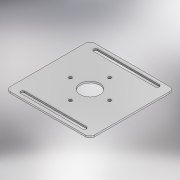
# Autodesk Inventor part: BaseTopPlate
Saved by Autodesk Inventor 2020.3 (Build 243373000, 373)
## iProperties
Created: 2021-08-02
Part Number: BaseTopPlate
Material: Aluminum
Document SubType Name: Modeling
Designer: justi
Density: 2.7 g/cm^3
Appearance: Aluminum - Polished
Author: justi
Autodesk Inventor part; units mm, degrees
ref_plane "YZ Plane" through (0, 0, 0) normal (1, 0, 0) x (0, 1, 0)
ref_plane "XZ Plane" through (0, 0, 0) normal (0, 1, 0) x (-1, 0, 0)
ref_plane "XY Plane" through (0, 0, 0) normal (0, 0, 1) x (1, 0, 0)
sketch "Sketch1" plane through (0, 0, 0) normal (0, 1, 0) x (-1, 0, 0)
  line L0 (-75, -75) -> (75, -75)
  line L1 (75, -75) -> (75, 75)
  line L2 (75, 75) -> (-75, 75)
  line L3 (-75, 75) -> (-75, -75)
  line L4 (-75, -75) -> (75, 75) construction
  line L5 (75, -75) -> (-75, 75) construction
  circle A0 centre (0, 0) radius 17.5
  line L6 (65, 65) -> (65, -65) construction
  line L7 (65, -65) -> (-65, -65) construction
  line L8 (-65, -65) -> (-65, 65) construction
  line L9 (-65, 65) -> (65, 65) construction
  line L10 (75, 65) -> (55, 65) construction
  line L11 (55, 65) -> (55, -65) construction
  line L12 (-75, 65) -> (-55, 65) construction
  line L13 (-55, 65) -> (-55, -65) construction
  line L14 (-55, 65) -> (55, 65) construction
  line L15 (-55, 61.43) -> (55, 61.43)
  line L16 (55, 68.57) -> (-55, 68.57)
  arc A1 (-55, 68.57) -> (-55, 61.43) centre (-55, 65) ccw
  arc A2 (55, 61.43) -> (55, 68.57) centre (55, 65) ccw
  line L17 (-55, -65) -> (55, -65) construction
  line L18 (-55, -68.57) -> (55, -68.57)
  line L19 (55, -61.43) -> (-55, -61.43)
  arc A3 (-55, -61.43) -> (-55, -68.57) centre (-55, -65) ccw
  arc A4 (55, -68.57) -> (55, -61.43) centre (55, -65) ccw
  point P0 (0, 65)
  point P1 (0, -65)
  dimension "d0" = 150
  dimension "d1" = 150
  dimension "d2" = 35
  dimension "d3" = 10
  dimension "d4" = 20
  dimension "d5" = 20
  dimension "d6" = 7.14
  dimension "d7" = 7.14
  constraints: 44 end point, 8 point on circle, 8 tangent, 7 point on line, 6 midpoint, 6 parallel, 5 centre point, 4 perpendicular, 2 collinear, 1 coincident, 1 horizontal, 3 other
  measures "d0" distance of L2.end L1.end
  measures "d1" distance of L1.end L0.end
  measures "d2" diameter of A0
  measures "d3" distance between parallel lines of L1 L6
  measures "d4" distance of L10.start L10.end
  measures "d5" distance of L12.start L12.end
  measures "d6" diameter of A2
  measures "d7" diameter of A4
extrude "Extrusion1" add sketch "Sketch1" along normal blind 3
sketch "Sketch2" plane through (0, 3, 0) normal (0, 1, 0) x (1, 0, 0)
  circle A0 centre (0, 0) radius 35 construction
  line L0 (0, 0) -> (35, 0) construction
  line L1 (35, 0) -> (0, 35) construction
  line L2 (0, 35) -> (-35, 0) construction
  line L3 (-35, 0) -> (0, -35) construction
  line L4 (0, -35) -> (35, 0) construction
  dimension "d21" = 70
  constraints: 10 end point, 4 coincident, 4 point on circle, 3 perpendicular, 1 centre point, 1 horizontal
  measures "d21" diameter of A0
hole "Hole1" at (0, 3, 35) at (35, 3, 0) at (0, 3, -35) at (-35, 3, 0) direction (0, -1, 0) diameter 5.5 end through all clearance for "Hex Head Bolt" size "M5" standard "Ansi Metric M Profile"
fillet "Fillet1" radius 8 4 edges at (-75, 1.5, -75) (-75, 1.5, 75) (75, 1.5, 75) (75, 1.5, -75)
body "Solid1"
